power_button_nut (Autodesk Fusion 360 design; units mm, degrees)
Autodesk Fusion 360 part; units mm, degrees
sketch "Sketch1" plane through (0, 0, 0) normal (0, 1, 0) x (1, 0, 0)
  circle A0 centre (0, 0) radius 7.75
  line L0 (0, 0) -> (0, -11)
  line L1 (0, 0) -> (0, 11)
  line L2 (0, -9.375) -> (-5.4127, -9.375)
  line L3 (-5.4127, -9.375) -> (-10.8253, 0)
  line L4 (-10.8253, 0) -> (-5.4127, 9.375)
  line L5 (-5.4127, 9.375) -> (0, 9.375)
  line L6 (0, 9.375) -> (5.4127, 9.375)
  line L7 (5.4127, 9.375) -> (10.8253, 0)
  line L8 (10.8253, 0) -> (5.4127, -9.375)
  line L9 (0, -9.375) -> (5.4127, -9.375)
  dimension "d1" = 15.5
  dimension "d2" = 11
  dimension "d3" = 11
  dimension "d4" = 18.75
  dimension "d5" = 9.375
  dimension "d6" = 9.375
  dimension "d7" = 9.375
  dimension "d11" = 120
  dimension "d12" = 120
  dimension "d13" = 9.375
  dimension "d14" = 9.375
  constraint coincident A0.centre L0.start
  constraint vertical L0
  constraint parallel L0 L1
  constraint coincident L0 L2.start
  constraint perpendicular L0 L2
  constraint coincident L1 L5.end
  constraint perpendicular L1 L5
  constraint perpendicular L1 L6
  constraint perpendicular L0 L9
  constraint parallel L4 L8
  constraint parallel L3 L7
  measures "d1" diameter of A0
  measures "d2" distance of A0.centre L1.end
  measures "d3" distance of A0.centre L0.end
  measures "d4" distance of L2 L5
  measures "d5" distance of A0.centre L5
  measures "d6" distance of A0.centre L4
  measures "d7" distance of A0.centre L3
  measures "d11" angle of L6 L7
  measures "d12" angle of L7 L8
  measures "d13" distance of A0.centre L7
  measures "d14" distance of A0.centre L8
extrude "Extrude1" add sketch "Sketch1" along normal blind 2.35 contours A0 L0 L1 L6 L7 L8 L9 | A0 L0 L1 L2 L3 L4 L5
equation "d3 = d2"
equation "d5 = ( 18.75 / 2 ) * 1 mm"
equation "d6 = d5"
equation "d7 = d5"
equation "d12 = d11"
equation "d13 = d5"
equation "d14 = d5"
